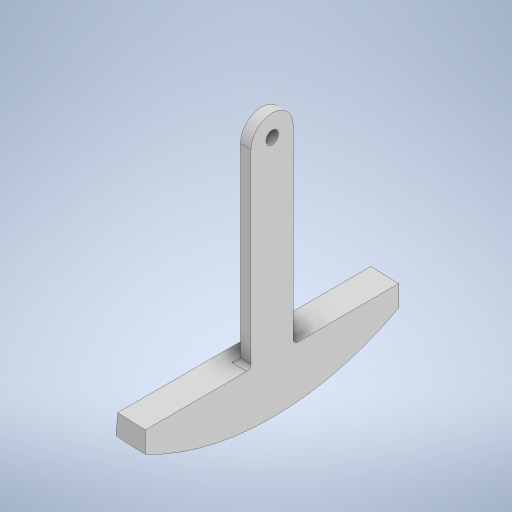
# Autodesk Inventor part: 受動歩行
Saved by Autodesk Inventor 2023 (Build 270158000, 158)
## iProperties
Created: 2024-05-29
Part Number: 受動歩行
Material: 一般
Document SubType Name: Modeling
Designer: babar
Density: 1 g/cm^3
Appearance: 既定
Author: babar
Autodesk Inventor part; units mm, degrees
ref_plane "YZ Plane" through (0, 0, 0) normal (1, 0, 0) x (0, 1, 0)
ref_plane "XZ Plane" through (0, 0, 0) normal (0, 1, 0) x (-1, 0, 0)
ref_plane "XY Plane" through (0, 0, 0) normal (0, 0, 1) x (1, 0, 0)
sketch "スケッチ2" plane through (0, 0, 0) normal (1, 0, 0) x (0, 1, 0)
  line L0 (0, 0) -> (0, -120)
  line L1 (0, -120) -> (-10, -120)
  line L2 (0, 0) -> (-10, 0)
  line L3 (0, -60) -> (-25, -60)
  arc A0 (-10, 0) -> (-10, -120) centre (102.5, -60) ccw
  line L4 (150, 222.8516) -> (150, -392.0935)
  dimension "d14" = 120
  dimension "d15" = 10
  dimension "d16" = 10
  dimension "d17" = 25
  dimension "d18" = 300
  constraints: 10 end point, 3 point on circle, 2 horizontal, 2 vertical, 1 centre point, 1 midpoint, 1 perpendicular
  measures "d14" distance of L0.start L0.end
  measures "d15" distance of L0.end L1.end
  measures "d16" distance of L0.start L2.end
  measures "d17" distance of L3.start L3.end
  measures "d18" diameter of L0 L4
revolve "回転2" add sketch "スケッチ2" angle 5 about axis through (0, 150, 222.8516) along (0, 0, -1)
sketch "スケッチ3" plane through (0, -10, -120) normal (1, 0, 0) x (0, 0, -1)
  line L0 (-70, 110) -> (-50, 110)
  line L1 (-50, 110) -> (-50, 10)
  line L2 (-50, 10) -> (-70, 10)
  line L3 (-70, 10) -> (-70, 110)
  line L4 (0, 0) -> (0, 10) projected
  line L5 (0, 10) -> (-120, 10) projected
  dimension "d20" = 100
  dimension "d21" = 20
  dimension "d22" = 50
  dimension "d23" = 0
  constraints: 8 end point, 2 parallel, 1 horizontal, 1 perpendicular
  measures "d20" distance of L0.end L1.end
  measures "d21" distance of L0.start L0.end
  measures "d22" distance between parallel lines of L4 L1
  measures "d23" distance between parallel lines of L5 L2
extrude "押し出し1" add sketch "スケッチ3" against normal blind 5
fillet "フィレット2" radius 2 3 edges at (-2.5003, 0.0208, -50) (-5, 0.0834, -60) (-2.5003, 0.0208, -70)
sketch "スケッチ4" plane through (0, -10, -120) normal (1, 0, 0) x (0, 0, -1)
  line L0 (-50, 12) -> (-50, 110) projected
  line L1 (-50, 110) -> (-70, 110) projected
  point P0 (-120, 10)
  point P1 (-60, 100)
  dimension "d27" = 10
  dimension "d28" = 10
  measures "d27" distance from line of L0 point (-60, 100)
  measures "d28" distance from line of L1 point (-60, 100)
hole "穴1" at (0, 90, -60) direction (-1, 0, 0) diameter 6 end through all
fillet "フィレット3" radius 10 2 edges at (-2.5, 100, -50) (-2.5, 100, -70)
